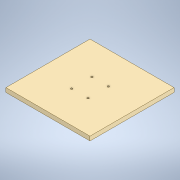
# Autodesk Inventor part: MDFTop
Saved by Autodesk Inventor 2022 (Build 260153000, 153)
## iProperties
Created: 2021-07-14
Part Number: MDFTop
Material: Generic
Document SubType Name: Modeling
Designer: BBL
Density: 1 g/cm^3
Appearance: Beige
Author: BBL
Autodesk Inventor part; units mm, degrees
ref_plane "YZ Plane" through (0, 0, 0) normal (1, 0, 0) x (0, 1, 0)
ref_plane "XZ Plane" through (0, 0, 0) normal (0, 1, 0) x (-1, 0, 0)
ref_plane "XY Plane" through (0, 0, 0) normal (0, 0, 1) x (1, 0, 0)
sketch "Sketch1" plane through (0, 0, 0) normal (0, 1, 0) x (-1, 0, 0)
  line L0 (-120, 120) -> (120, 120)
  line L1 (120, 120) -> (120, -120)
  line L2 (120, -120) -> (-120, -120)
  line L3 (-120, -120) -> (-120, 120)
  line L4 (-120, 120) -> (120, -120) construction
  line L5 (120, 120) -> (-120, -120) construction
  circle A0 centre (23.5, 29) radius 2.75
  circle A1 centre (23.5, -29) radius 2.75
  circle A2 centre (-23.5, 29) radius 2.75
  circle A3 centre (-23.5, -29) radius 2.75
  point P0 (0, 0)
  dimension "d0" = 240
  dimension "d1" = 240
  dimension "d4" = 5.5
  dimension "d7" = 58
  dimension "d10" = 47
  dimension "d13" = 29
  dimension "d14" = 29
  dimension "d15" = 23.5
  dimension "d16" = 23.5
  constraints: 12 end point, 4 centre point, 2 horizontal, 2 midpoint, 2 parallel, 1 perpendicular, 1 vertical, 6 other
  measures "d0" distance of L1.end L2.end
  measures "d1" distance of L0.end L1.end
  measures "d4" diameter of A0
  measures "d7" distance of A0.centre A1.centre
  measures "d10" distance of A0.centre A2.centre
  measures "d13" vertical distance of point (0, 0) A0.centre
  measures "d14" vertical distance of A1.centre point (0, 0)
  measures "d15" horizontal distance of point (0, 0) A0.centre
  measures "d16" horizontal distance of point (0, 0) A2.centre
extrude "Extrusion1" add sketch "Sketch1" along normal blind 12
equation "\"d13\" = d14"
equation "\"d15\" = d16"
body "Solid1"
